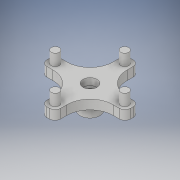
# Autodesk Inventor part: planetaryGearMt2
Saved by Autodesk Inventor 2019 (Build 230136000, 136)
## iProperties
Created: 2019-10-26
Part Number: planetaryGearMt2
Material: Generic
Document SubType Name: Modeling
Designer: test
Density: 1 g/cm^3
Appearance: Default
Author: test
Autodesk Inventor part; units mm, degrees
ref_plane "YZ Plane" through (0, 0, 0) normal (1, 0, 0) x (0, 1, 0)
ref_plane "XZ Plane" through (0, 0, 0) normal (0, 1, 0) x (-1, 0, 0)
ref_plane "XY Plane" through (0, 0, 0) normal (0, 0, 1) x (1, 0, 0)
sketch "Sketch1" plane through (0, 0, 0) normal (0, 1, 0) x (-1, 0, 0)
  circle A0 centre (0, 19.05) radius 2.2225
  circle A1 centre (-19.05, 0) radius 2.2225
  circle A2 centre (0, -19.05) radius 2.2225
  circle A3 centre (19.05, 0) radius 2.2225
  line L0 (0.635, 24.639) -> (0, 24.639)
  line L1 (0, 0) -> (0, 2.5439)
  line L2 (3.81, -19.812) -> (3.81, -16.51)
  line L3 (3.81, 16.51) -> (3.81, 19.812)
  line L4 (-19.812, 3.81) -> (-16.51, 3.81)
  line L5 (16.51, 3.81) -> (19.812, 3.81)
  line L6 (-3.81, 19.812) -> (-3.81, 16.51)
  line L7 (-3.81, -16.51) -> (-3.81, -19.812)
  line L8 (19.812, -3.81) -> (16.51, -3.81)
  line L9 (-16.51, -3.81) -> (-19.812, -3.81)
  arc A4 (3.81, 16.51) -> (16.51, 3.81) centre (16.51, 16.51) ccw
  arc A5 (16.51, -3.81) -> (3.81, -16.51) centre (16.51, -16.51) ccw
  arc A6 (-16.51, 3.81) -> (-3.81, 16.51) centre (-16.51, 16.51) ccw
  arc A7 (-3.81, -16.51) -> (-16.51, -3.81) centre (-16.51, -16.51) ccw
  line L10 (0, -3.81) -> (0, 0)
  line L11 (0, 3.81) -> (0, 0)
  line L12 (3.81, -19.812) -> (3.81, -16.51)
  line L13 (16.51, 3.81) -> (19.812, 3.81)
  line L14 (21.2725, 0) -> (16.8275, 0)
  line L15 (19.812, 3.81) -> (16.51, 3.81)
  line L16 (19.812, -3.81) -> (16.51, -3.81)
  line L17 (0, -3.81) -> (0.635, -3.81)
  line L18 (16.51, -3.81) -> (19.812, -3.81)
  line L19 (-19.812, -3.81) -> (-16.51, -3.81)
  line L20 (-3.81, -16.51) -> (-3.81, -19.812)
  line L21 (-3.81, -19.812) -> (-3.81, -16.51)
  line L22 (0, 0) -> (0.635, 0)
  line L23 (-0.635, 24.639) -> (0.635, 24.639)
  line L24 (0.635, 0) -> (0, 0)
  line L25 (-3.81, 16.51) -> (-3.81, 19.812)
  line L26 (22.987, -0.635) -> (22.987, 0.635)
  arc A8 (-24.0273, 24.8189) -> (-24.2117, 24.639) centre (0, 0) ccw
  line L27 (-19.812, 3.81) -> (-16.51, 3.81)
  line L28 (-3.81, 19.812) -> (-3.81, 16.51)
  line L29 (3.81, 19.812) -> (3.81, 16.51)
  line L30 (3.81, 19.812) -> (3.81, 16.51)
  line L31 (19.812, 3.81) -> (16.51, 3.81)
  line L32 (16.51, -3.81) -> (19.812, -3.81)
  line L33 (3.81, -16.51) -> (3.81, -19.812)
  line L34 (-19.812, -3.81) -> (-16.51, -3.81)
  line L35 (0, -3.81) -> (0.635, -3.81)
  line L36 (0.635, 3.81) -> (0, 3.81)
  line L37 (-16.51, 3.81) -> (-19.812, 3.81)
  arc A9 (19.812, -3.81) -> (22.987, -0.635) centre (19.812, -0.635) ccw
  arc A10 (22.987, 0.635) -> (19.812, 3.81) centre (19.812, 0.635) ccw
  line L38 (0, 0) -> (7.5297, 7.5297)
  line L39 (0, 0) -> (7.5297, -7.5297)
  circle A11 centre (0, 19.05) radius 2.2225
  line L40 (3.81, 16.51) -> (3.81, 19.812)
  line L41 (-3.81, 19.812) -> (-3.81, 16.51)
  line L42 (3.81, 16.51) -> (3.81, 19.812)
  line L43 (3.81, 19.812) -> (3.81, 16.51)
  line L44 (3.81, 19.812) -> (3.81, 16.51)
  line L45 (-3.81, 19.812) -> (-3.81, 16.51)
  line L46 (-3.81, 16.51) -> (-3.81, 19.812)
  line L47 (-3.81, 16.51) -> (-3.81, 19.812)
  line L48 (0, 21.2725) -> (0, 16.8275)
  arc A12 (-0.635, 22.987) -> (-3.81, 19.812) centre (-0.635, 19.812) ccw
  line L49 (-0.635, 22.987) -> (0.635, 22.987)
  arc A13 (3.81, 19.812) -> (0.635, 22.987) centre (0.635, 19.812) ccw
  arc A14 (3.81, 16.51) -> (16.51, 3.81) centre (16.51, 16.51) ccw
  arc A15 (-16.51, 3.81) -> (-3.81, 16.51) centre (-16.51, 16.51) ccw
  arc A16 (-16.51, 3.81) -> (-3.81, 16.51) centre (-16.51, 16.51) ccw
  line L50 (-3.81, 16.51) -> (-3.81, 19.812)
  arc A17 (-0.635, 22.987) -> (-3.81, 19.812) centre (-0.635, 19.812) ccw
  arc A18 (3.81, 19.812) -> (0.635, 22.987) centre (0.635, 19.812) ccw
  line L51 (0.635, 22.987) -> (-0.635, 22.987)
  arc A19 (3.81, 16.51) -> (16.51, 3.81) centre (16.51, 16.51) ccw
  line L52 (3.81, 19.812) -> (3.81, 16.51)
  arc A20 (-3.81, -16.51) -> (-16.51, -3.81) centre (-16.51, -16.51) ccw
  line L53 (-16.51, -3.81) -> (-19.812, -3.81)
  arc A21 (-22.987, -0.635) -> (-19.812, -3.81) centre (-19.812, -0.635) ccw
  arc A22 (-19.812, 3.81) -> (-22.987, 0.635) centre (-19.812, 0.635) ccw
  line L54 (-22.987, 0.635) -> (-22.987, -0.635)
  arc A23 (-16.51, 3.81) -> (-3.81, 16.51) centre (-16.51, 16.51) ccw
  line L55 (-19.812, 3.81) -> (-16.51, 3.81)
  arc A24 (16.51, -3.81) -> (3.81, -16.51) centre (16.51, -16.51) ccw
  line L56 (3.81, -16.51) -> (3.81, -19.812)
  arc A25 (0.635, -22.987) -> (3.81, -19.812) centre (0.635, -19.812) ccw
  arc A26 (-3.81, -19.812) -> (-0.635, -22.987) centre (-0.635, -19.812) ccw
  line L57 (-0.635, -22.987) -> (0.635, -22.987)
  arc A27 (-3.81, -16.51) -> (-16.51, -3.81) centre (-16.51, -16.51) ccw
  line L58 (-3.81, -19.812) -> (-3.81, -16.51)
  point P0 (19.05, 0)
  point P1 (0, -19.05)
  point P2 (-2.9852, -22.987)
  point P3 (-3.81, -29.2166)
  point P4 (0, 34.544)
  point P5 (-24.0273, 0)
  point P6 (0, -24.0273)
  point P7 (0, 19.05)
  point P8 (-7.5297, 7.5297)
  point P9 (7.5297, 7.5297)
  point P10 (-7.5297, -7.5297)
  point P11 (-7.5297, 7.5297)
  point P12 (7.5297, -7.5297)
  point P13 (-7.5297, -7.5297)
  dimension "d4" = 360
  dimension "d5" = 4.445
  dimension "d6" = 360
  dimension "d7" = 3.175
  dimension "d16" = 360
  constraints: 118 end point, 52 point on circle, 28 centre point, 15 parallel, 13 symmetric about line, 12 tangent, 9 point on line, 7 horizontal, 4 equal radius, 4 perpendicular, 1 coincident, 1 vertical, 104 other
  measures "d5" diameter of A0
  measures "d7" radius of A9
extrude "Extrusion1" add sketch "Sketch1" along normal blind 5.08
extrude "Extrusion2" add sketch "Sketch1" along normal blind 11.43 contours A0 L48 | L48 A0 | A1 | A2 | A3 L14 picked at (18.3725, -0.5216)
extrude "Extrusion3" add sketch "Sketch1" along normal blind 11.43 contours L14 A3 picked at (19.7275, 0.5216)
sketch "Sketch2" plane through (0, 5.08, 0) normal (0, 1, 0) x (1, 0, 0)
  circle A0 centre (0, 0) radius 2.8575
  dimension "d18" = 5.715
  constraints: 1 centre point, 1 coincident
  measures "d18" diameter of A0
extrude "Extrusion4" cut sketch "Sketch2" against normal blind 11.43
sketch "Sketch3" plane through (0, 0, 0) normal (0, -1, 0) x (1, 0, 0)
  circle A0 centre (0, 0) radius 2.8575
  circle A1 centre (0, 0) radius 5.3975
  dimension "d21" = 2.54
  dimension "d22" = 5.715
  constraints: 2 centre point, 2 coincident
  measures "d21" radial gap between concentric circles of A1 A0
  measures "d22" diameter of A0
extrude "Extrusion5" add sketch "Sketch3" along normal blind 5.08
sketch "Sketch4" plane through (0, 5.08, 0) normal (0, 1, 0) x (1, 0, 0)
  circle A0 centre (0, 0) radius 3.81
  dimension "d25" = 7.62
  constraints: 1 centre point, 1 coincident
  measures "d25" diameter of A0
extrude "Extrusion6" cut sketch "Sketch4" against normal blind 3.81
sketch "Sketch5" plane through (0, 1.27, 0) normal (0, 1, 0) x (1, 0, 0)
  circle A0 centre (0, 0) radius 3.175
  dimension "d28" = 6.35
  constraints: 1 centre point, 1 coincident
  measures "d28" diameter of A0
extrude "Extrusion7" cut sketch "Sketch5" against normal blind 50.8
sketch "Sketch6" plane through (0, 1.27, 0) normal (0, 1, 0) x (1, 0, 0)
  circle A0 centre (0, 0) radius 1.905
  circle A1 centre (0, 0) radius 3.175
  dimension "d31" = 3.81
  constraints: 2 centre point, 2 coincident
  measures "d31" diameter of A0
extrude "Extrusion8" add sketch "Sketch6" against normal blind 2.54
sketch "Sketch7" plane through (0, -5.08, 0) normal (0, -1, 0) x (1, 0, 0)
  circle A0 centre (0, 0) radius 3.175
  circle A1 centre (0, 0) radius 5.3975
  constraints: 2 centre point, 2 coincident
extrude "Extrusion9" add sketch "Sketch7" along normal blind 2.54
body "Solid1"
